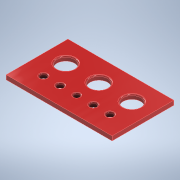
# Autodesk Inventor part: plateForFileSet
Saved by Autodesk Inventor 2021 (Build 250183000, 183)
## iProperties
Created: 2020-03-12
Part Number: plateForFileSet
Material: PET Plastic
Document SubType Name: Modeling
Designer: robst
Density: 1.541 g/cm^3
Appearance: Red
Author: robst
Autodesk Inventor part; units mm, degrees
ref_plane "YZ Plane" through (0, 0, 0) normal (1, 0, 0) x (0, 1, 0)
ref_plane "XZ Plane" through (0, 0, 0) normal (0, 1, 0) x (-1, 0, 0)
ref_plane "XY Plane" through (0, 0, 0) normal (0, 0, 1) x (1, 0, 0)
sketch "Sketch1" plane through (0, 0, 0) normal (0, 1, 0) x (-1, 0, 0)
  line L0 (76.2, 44.45) -> (-76.2, 44.45)
  line L1 (-76.2, 44.45) -> (-76.2, -44.45)
  line L2 (-76.2, -44.45) -> (76.2, -44.45)
  line L3 (76.2, -44.45) -> (76.2, 44.45)
  line L4 (76.2, 44.45) -> (-76.2, -44.45) construction
  line L5 (-76.2, 44.45) -> (76.2, -44.45) construction
  point P0 (0, 0)
  dimension "depth" = 88.9
  dimension "width" = 152.4
  constraints: 12 end point, 2 midpoint, 2 parallel, 1 horizontal, 1 perpendicular
  measures "depth" distance of L2.end L0.start
  measures "width" distance of L1.end L2.end
extrude "Extrusion1" add sketch "Sketch1" against normal blind 6.35
sketch "Sketch4" plane through (0, 0, 0) normal (0, 1, 0) x (1, 0, 0)
  line L0 (-76.2, -44.45) -> (-76.2, 44.45) construction
  line L1 (-76.2, -19.05) -> (76.2, -19.05) construction
  line L2 (76.2, 44.45) -> (76.2, -44.45) construction
  line L3 (-76.2, -44.45) -> (76.2, -44.45) projected
  circle A0 centre (-48.006, -19.05) radius 4.445
  circle A1 centre (-24.0574, -19.05) radius 4.445
  circle A2 centre (-0.1089, -19.05) radius 3.81
  circle A3 centre (23.8397, -19.05) radius 4.445
  circle A4 centre (47.7883, -19.05) radius 4.445
  line L4 (-76.2, 12.7) -> (76.2, 12.7) construction
  circle A5 centre (-47.625, 12.7) radius 12.7
  circle A6 centre (0, 12.7) radius 12.7
  circle A7 centre (47.625, 12.7) radius 12.7
  point P0 (0, 0)
  dimension "d16" = 25.4
  dimension "file1Hole" = 8.89
  dimension "gap0" = 23.749
  dimension "file2Hole" = 8.89
  dimension "gap1" = 23.9486
  dimension "file3Hole" = 7.62
  dimension "gap2" = 23.9486
  dimension "gap3" = 23.9486
  dimension "gap4" = 23.9486
  dimension "file4Hole" = 8.89
  dimension "file5Hole" = 8.89
  dimension "d27" = 23.9667
  dimension "frontToBackRowGap" = 31.75
  dimension "file7Hole" = 25.4
  dimension "file8Hole" = 25.4
  dimension "gap7" = 47.625
  dimension "file9Hole" = 25.4
  dimension "gap8" = 47.625
  dimension "gap6" = 28.575
  dimension "d53" = 28.575
  constraints: 11 point on line, 8 centre point, 4 end point, 1 horizontal, 1 midpoint, 1 perpendicular
  measures "d16" distance between parallel lines of L1 L3
  measures "file1Hole" diameter of A0
  measures "gap0" distance edge to line of A0 L0
  measures "file2Hole" diameter of A1
  measures "gap1" distance of A1.centre A0.centre
  measures "file3Hole" diameter of A2
  measures "gap2" distance of A2.centre A1.centre
  measures "gap3" distance of A3.centre A2.centre
  measures "gap4" distance of A4.centre A3.centre
  measures "file4Hole" diameter of A3
  measures "file5Hole" diameter of A4
  measures "d27" distance edge to line of A4 L2
  measures "frontToBackRowGap" distance between parallel lines of L4 L1
  measures "file7Hole" diameter of A5
  measures "file8Hole" diameter of A6
  measures "gap7" distance of A6.centre A5.centre
  measures "file9Hole" diameter of A7
  measures "gap8" distance of A7.centre A6.centre
  measures "gap6" distance from line of A5.centre L0
  measures "d53" distance from line of A7.centre L2
extrude "Extrusion3" cut sketch "Sketch4" against normal through all
fillet "Fillet4" radius 1.5875 8 edges at (-60.325, 0, -12.7) (-12.7, 0, -12.7) (34.925, 0, -12.7) (43.3433, 0, 19.05) (19.3947, 0, 19.05) (-3.9189, 0, 19.05) (-28.5024, 0, 19.05) (-52.451, 0, 19.05)
equation "\"frontGapBetweenHoles\" = 8.70857"
equation "\"backGapBetweenHoles\" = 9.525"
equation "\"centerLineForFrontText\" = 8.3185"
equation "\"centerLineForBackText\" = 40.64"
equation "\"largeFileHoleDiameter\" = 25.4"
equation "\"smallFileHoleDiameter\" = 8.89"
equation "\"filesInBackRow\" = 76.2"
equation "\"filesInFrontRow\" = 177.8"
equation "\"largeFileHandleDiameter\" = 38.1"
equation "\"smallFileHandleDiameter\" = 15.24"
body "Solid1"
